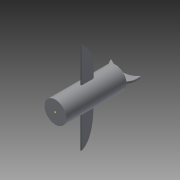
# Autodesk Inventor part: wings
Saved by Autodesk Inventor 2015 SP1 (Build 190203100, 203)
## iProperties
Created: 2018-02-27
Part Number: wings
Material: Generic
Document SubType Name: Modeling
Designer: 325609
Density: 1 g/cm^3
Appearance: Default
Author: 325609
Autodesk Inventor part; units mm, degrees
ref_plane "YZ Plane" through (0, 0, 0) normal (1, 0, 0) x (0, 1, 0)
ref_plane "XZ Plane" through (0, 0, 0) normal (0, 1, 0) x (-1, 0, 0)
ref_plane "XY Plane" through (0, 0, 0) normal (0, 0, 1) x (1, 0, 0)
sketch "Sketch1" plane through (0, 0, 0) normal (0, 0, 1) x (1, 0, 0)
  circle A0 centre (0, 0) radius 39.4843
  dimension "d0" = 78.9686
  constraints: 1 centre point, 1 coincident
  measures "d0" diameter of A0
extrude "Extrusion1" add sketch "Sketch1" along normal blind 218.44
sketch "Sketch2" plane through (0, 0, 0) normal (1, 0, 0) x (0, 1, 0)
  line L0 (39.4843, 0) -> (39.4843, 218.44)
  line L1 (39.4843, 83.5771) -> (39.4843, 128.0271)
  line L2 (39.4843, 128.0271) -> (166.4843, 128.0271)
  line L3 (166.4843, 128.0271) -> (131.3819, 76.4226) construction
  line L4 (131.3819, 76.4226) -> (39.4843, 83.5771) construction
  spline S0 degree 2 poles (166.4843, 128.0271) (131.3819, 76.4226) (39.4843, 83.5771) knots 1 1 1 2 2 2
  line L5 (-39.4843, 83.5747) -> (-39.4843, 128.0271)
  line L6 (-39.4843, 0) -> (-39.4843, 218.44) projected
  line L7 (-39.4843, 83.5747) -> (-39.4843, 128.0271)
  line L8 (-39.4843, 128.0271) -> (-166.4843, 128.0271)
  line L9 (-166.4843, 128.0271) -> (-149.7384, 83.5714) construction
  line L10 (-149.7384, 83.5714) -> (-39.4843, 83.5747) construction
  spline S1 degree 2 poles (-166.4843, 128.0271) (-149.7384, 83.5714) (-39.4843, 83.5747) knots 1 1 1 2 2 2
  line L11 (-39.4843, 128.0271) -> (48.468, 128.0271)
  line L12 (-39.4843, 83.5747) -> (39.4843, 83.5771)
  line L13 (-54.9885, 128.0271) -> (39.4843, 128.0271)
  line L14 (39.4843, 0) -> (39.4843, 218.44) projected
  line L15 (-39.4843, 83.5747) -> (39.4843, 83.5771)
  point P0 (0, 0)
  dimension "d3" = 44.45
  dimension "d4" = 127
  dimension "d5" = 127
  constraints: 20 end point, 7 point on line, 3 perpendicular, 1 collinear, 8 other
  measures "d3" distance of L1.start L1.end
  measures "d4" distance of L1.end L2.end
  measures "d5" distance of L5.end L8.end
extrude "Extrusion2" add sketch "Sketch2" along normal blind 3.175
chamfer "Chamfer1" distance 3.175 angle 45 1 edges at (3.175, -102.9204, 128.0271)
chamfer "Chamfer2" distance 3.175 angle 45 1 edges at (3.175, 102.9204, 128.0271)
sketch "Sketch3" plane through (0, 0, 0) normal (0, 1, 0) x (-1, 0, 0)
  line L0 (-39.4843, 0) -> (39.4843, 0) projected
  line L1 (-33.3888, 0) -> (9.1562, 0)
  line L2 (9.1562, 0) -> (44.2001, -3.3503) construction
  line L3 (44.2001, -3.3503) -> (62.7444, -45.9959) construction
  spline S0 degree 2 poles (9.1562, 0) (44.2001, -3.3503) (62.7444, -45.9959) knots 1 1 1 2 2 2
  line L4 (62.7444, -45.9959) -> (-9.2544, -6.0902) construction
  line L5 (-9.2544, -6.0902) -> (-44.8829, -45.9959) construction
  spline S1 degree 2 poles (62.7444, -45.9959) (-9.2544, -6.0902) (-44.8829, -45.9959) knots 1 1 1 2 2 2
  line L6 (-44.8829, -45.9959) -> (-49.2667, -15.2331) construction
  line L7 (-49.2667, -15.2331) -> (-33.3888, 0) construction
  spline S2 degree 2 poles (-44.8829, -45.9959) (-49.2667, -15.2331) (-33.3888, 0) knots 1 1 1 2 2 2
  point P0 (0, 0)
  dimension "d14" = 42.545
  constraints: 2 end point, 2 point on line, 9 other
  measures "d14" distance of L1.start L1.end
extrude "Extrusion3" add sketch "Sketch3" along normal mid plane 6.35
fillet "Fillet1" radius 3.175 1 edges at (12.1163, 3.175, 0)
fillet "Fillet2" radius 3.175 1 edges at (12.1163, -3.175, 0)
sketch "Sketch4" plane through (0, 0, 218.44) normal (0, 0, 1) x (1, 0, 0)
  point P0 (0, 0)
body "Solid1"
